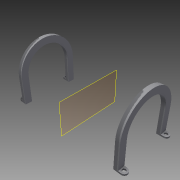
# Autodesk Inventor part: handle_it
Saved by Autodesk Inventor 2014 (Build 180170000, 170)
## iProperties
Created: 2013-09-16
Part Number: handle_it
Material: Generic
Document SubType Name: Modeling
Designer: Nick
Density: 1 g/cm^3
Appearance: Default
Author: Nick
Autodesk Inventor part; units mm, degrees
ref_plane "XZ Plane" through (0, 0, 0) normal (0, 1, 0) x (-1, 0, 0)
ref_plane "XY Plane" through (0, 0, 0) normal (0, 0, 1) x (1, 0, 0)
sketch "Sketch1" plane through (0, 0, 0) normal (0, 0, 1) x (1, 0, 0)
  circle A0 centre (0, 30) radius 2
  circle A1 centre (0, 30) radius 4
  line L0 (0, 26) -> (8, 26)
  line L1 (8, 26) -> (8, 34)
  line L2 (8, 34) -> (0, 34)
  point P0 (0, 0)
  dimension "d0" = 2
  dimension "d2" = 4
  dimension "d6" = 30
  dimension "d7" = 8
  constraints: 6 end point, 2 centre point, 2 perpendicular, 2 point on circle, 2 tangent, 1 coincident, 1 horizontal, 1 vertical alignment
  measures "d0" radial gap between concentric circles of A1 A0
  measures "d2" diameter of A0
  measures "d6" distance of point (0, 0) A0.centre
  measures "d7" distance of L1.end L2.end
extrude "Extrusion1" add sketch "Sketch1" along normal blind 2
sketch "Sketch2" plane through (0, 0, 2) normal (0, 0, 1) x (1, 0, 0)
  line L0 (0, 26) -> (8, 26) projected
  line L1 (8, 26) -> (8, 34) projected
  line L2 (8, 34) -> (0, 34) projected
  line L3 (3, 26) -> (3, 34)
  line L4 (-6.4, 0) -> (10.4, 0) projected
  point P0 (0, 0)
  dimension "d10" = 5
  constraints: 2 end point, 2 point on line, 1 perpendicular
  measures "d10" distance between parallel lines of L1 L3
extrude "Extrusion2" add sketch "Sketch2" along normal blind 30
mirror "Mirror1" about plane through (0, 0, 0) normal (0, 1, 0) of "Extrusion1", "Extrusion2"
sketch "RevolutionSketch" plane through (0, 0, 32) normal (0, 0, 1) x (1, 0, 0)
  line L0 (3, 26) -> (8, 26) projected
  line L1 (8, 26) -> (8, 34) projected
  line L2 (8, 34) -> (3, 34) projected
  line L3 (3, 34) -> (3, 26) projected
  line L4 (-6.4, 0) -> (10.4, 0) projected
  point P0 (0, 0)
revolve "Revolution2" add sketch "RevolutionSketch" angle 180 about axis through (-10, 0, 32) along (1, 0, 0)
ref_plane "Work Plane1" through (69, 0, 0) normal (1, 0, 0) x (0, 1, 0)
mirror "Mirror2" about plane through (69, 0, 0) normal (1, 0, 0) of "Extrusion1", "Mirror1", "Extrusion2", "Revolution2"
body "Solid1"
